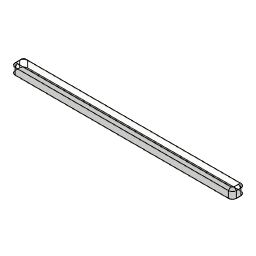
Rubber Foot v4 (Autodesk Fusion 360 design; units mm, degrees)
Autodesk Fusion 360 part; units mm, degrees
sketch "Foot Outline" plane through (0, 0, 0) normal (0, 1, 0) x (1, 0, 0)
  line L0 (48, 3) -> (-48, 3)
  line L1 (-50, 1) -> (-50, -1)
  line L2 (-48, -3) -> (48, -3)
  line L3 (50, -1) -> (50, 1)
  line L4 (50, 3) -> (-50, -3) construction
  line L5 (-50, 3) -> (50, -3) construction
  arc A0 (-50, -1) -> (-48, -3) centre (-48, -1) ccw
  arc A1 (-48, 3) -> (-50, 1) centre (-48, 1) ccw
  arc A2 (50, 1) -> (48, 3) centre (48, 1) ccw
  arc A3 (48, -3) -> (50, -1) centre (48, -1) ccw
  arc A4 (-49.8, -1) -> (-48, -2.8) centre (-48, -1) ccw
  line L6 (-48, -2.8) -> (48, -2.8)
  arc A5 (48, -2.8) -> (49.8, -1) centre (48, -1) ccw
  line L7 (49.8, -1) -> (49.8, 1)
  arc A6 (49.8, 1) -> (48, 2.8) centre (48, 1) ccw
  line L8 (48, 2.8) -> (-48, 2.8)
  arc A7 (-48, 2.8) -> (-49.8, 1) centre (-48, 1) ccw
  line L9 (-49.8, 1) -> (-49.8, -1)
  dimension "d1" = 100
  dimension "d2" = 6
  dimension "d3" = 2
  dimension "d4" = 2
  dimension "d5" = 2
  dimension "d9" = -0.2
  constraint horizontal L0
  constraint perpendicular L0 L1
  constraint parallel L0 L2
  constraint parallel L1 L3
  constraint coincident L4 origin
  constraint coincident L5 origin
  constraint coincident L4.end L2
  constraint coincident L4.end L1
  constraint tangent L2 A0
  constraint tangent L1 A0
  constraint coincident L5.start L1
  constraint coincident L5.start L0
  constraint tangent L1 A1
  constraint tangent L0 A1
  constraint coincident L4.start L0
  constraint coincident L4.start L3
  constraint tangent L0 A2
  constraint tangent L3 A2
  constraint coincident L5.end L3
  constraint coincident L5.end L2
  constraint tangent L3 A3
  constraint tangent L2 A3
  constraint equal A2 A3
  measures "d1" distance of L4.end L5.end
  measures "d2" distance of L5.start L4.end
  measures "d3" radius of A0
  measures "d4" radius of A1
  measures "d5" radius of A2
extrude "Extrude2" add sketch "Foot Outline" along normal blind 4 contours A4 L6 A5 L7 A6 L8 A7 L9
chamfer "Chamfer2" distance 1 angle 45 8 edges at (0, 4, 2.8) (49.2728, 4, 2.2728) (49.8, 4, 0) (49.2728, 4, -2.2728) (0, 4, -2.8) (-49.2728, 4, -2.2728) (-49.8, 4, 0) (-49.2728, 4, 2.2728)
named bodies: "Foot"
